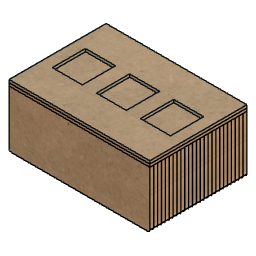
speacker-prototype1 (Autodesk Fusion 360 design; units mm, degrees)
Autodesk Fusion 360 part; units mm, degrees
(part 1 of 2)
sketch "スケッチ1" plane through (0, 0, 0) normal (0, 1, 0) x (1, 0, 0)
  line L0 (3, 0) -> (196.5, 0)
  line L1 (199.5, -3) -> (199.5, -80)
  line L2 (199.5, -80) -> (0, -80)
  line L3 (0, -80) -> (0, -3)
  arc A0 (3, 0) -> (0, -3) centre (3, -3) ccw
  arc A1 (199.5, -3) -> (196.5, 0) centre (196.5, -3) ccw
  line L4 (3, -74) -> (3, -6)
  line L5 (193.5, -77) -> (6, -77)
  line L6 (196.5, -6) -> (196.5, -74)
  line L7 (6, -3) -> (193.5, -3)
  arc A2 (3, -74) -> (6, -77) centre (6, -74) ccw
  arc A3 (6, -3) -> (3, -6) centre (6, -6) ccw
  arc A4 (193.5, -77) -> (196.5, -74) centre (193.5, -74) ccw
  arc A5 (196.5, -6) -> (193.5, -3) centre (193.5, -6) ccw
  line L8 (190.5, -74) -> (9, -74)
  line L9 (193.5, -9) -> (193.5, -71)
  line L10 (9, -6) -> (190.5, -6)
  line L11 (6, -71) -> (6, -9)
  arc A6 (6, -71) -> (9, -74) centre (9, -71) ccw
  arc A7 (9, -6) -> (6, -9) centre (9, -9) ccw
  arc A8 (193.5, -9) -> (190.5, -6) centre (190.5, -9) ccw
  arc A9 (190.5, -74) -> (193.5, -71) centre (190.5, -71) ccw
  line L12 (187.5, -71) -> (12, -71)
  line L13 (190.5, -12) -> (190.5, -68)
  line L14 (12, -9) -> (187.5, -9)
  line L15 (9, -68) -> (9, -12)
  arc A10 (9, -68) -> (12, -71) centre (12, -68) ccw
  arc A11 (12, -9) -> (9, -12) centre (12, -12) ccw
  arc A12 (187.5, -71) -> (190.5, -68) centre (187.5, -68) ccw
  arc A13 (190.5, -12) -> (187.5, -9) centre (187.5, -12) ccw
  line L16 (184.5, -68) -> (15, -68)
  line L17 (187.5, -15) -> (187.5, -65)
  line L18 (15, -12) -> (184.5, -12)
  line L19 (12, -65) -> (12, -15)
  arc A14 (12, -65) -> (15, -68) centre (15, -65) ccw
  arc A15 (15, -12) -> (12, -15) centre (15, -15) ccw
  arc A16 (184.5, -68) -> (187.5, -65) centre (184.5, -65) ccw
  arc A17 (187.5, -15) -> (184.5, -12) centre (184.5, -15) ccw
  line L20 (181.5, -65) -> (18, -65)
  line L21 (184.5, -18) -> (184.5, -62)
  line L22 (18, -15) -> (181.5, -15)
  line L23 (15, -62) -> (15, -18)
  arc A18 (15, -62) -> (18, -65) centre (18, -62) ccw
  arc A19 (18, -15) -> (15, -18) centre (18, -18) ccw
  arc A20 (181.5, -65) -> (184.5, -62) centre (181.5, -62) ccw
  arc A21 (184.5, -18) -> (181.5, -15) centre (181.5, -18) ccw
  line L24 (178.5, -62) -> (21, -62)
  line L25 (181.5, -21) -> (181.5, -59)
  line L26 (21, -18) -> (178.5, -18)
  line L27 (18, -59) -> (18, -21)
  arc A22 (18, -59) -> (21, -62) centre (21, -59) ccw
  arc A23 (21, -18) -> (18, -21) centre (21, -21) ccw
  arc A24 (178.5, -62) -> (181.5, -59) centre (178.5, -59) ccw
  arc A25 (181.5, -21) -> (178.5, -18) centre (178.5, -21) ccw
  line L28 (175.5, -59) -> (24, -59)
  line L29 (178.5, -24) -> (178.5, -56)
  line L30 (24, -21) -> (175.5, -21)
  line L31 (21, -56) -> (21, -24)
  arc A26 (21, -56) -> (24, -59) centre (24, -56) ccw
  arc A27 (24, -21) -> (21, -24) centre (24, -24) ccw
  arc A28 (175.5, -59) -> (178.5, -56) centre (175.5, -56) ccw
  arc A29 (178.5, -24) -> (175.5, -21) centre (175.5, -24) ccw
  line L32 (172.5, -56) -> (27, -56)
  line L33 (175.5, -27) -> (175.5, -53)
  line L34 (27, -24) -> (172.5, -24)
  line L35 (24, -53) -> (24, -27)
  arc A30 (24, -53) -> (27, -56) centre (27, -53) ccw
  arc A31 (27, -24) -> (24, -27) centre (27, -27) ccw
  arc A32 (172.5, -56) -> (175.5, -53) centre (172.5, -53) ccw
  arc A33 (175.5, -27) -> (172.5, -24) centre (172.5, -27) ccw
  line L36 (169.5, -53) -> (30, -53)
  line L37 (172.5, -30) -> (172.5, -50)
  line L38 (30, -27) -> (169.5, -27)
  line L39 (27, -50) -> (27, -30)
  arc A34 (27, -50) -> (30, -53) centre (30, -50) ccw
  arc A35 (30, -27) -> (27, -30) centre (30, -30) ccw
  arc A36 (169.5, -53) -> (172.5, -50) centre (169.5, -50) ccw
  arc A37 (172.5, -30) -> (169.5, -27) centre (169.5, -30) ccw
  line L40 (166.5, -50) -> (33, -50)
  line L41 (169.5, -33) -> (169.5, -47)
  line L42 (33, -30) -> (166.5, -30)
  line L43 (30, -47) -> (30, -33)
  arc A38 (30, -47) -> (33, -50) centre (33, -47) ccw
  arc A39 (33, -30) -> (30, -33) centre (33, -33) ccw
  arc A40 (166.5, -50) -> (169.5, -47) centre (166.5, -47) ccw
  arc A41 (169.5, -33) -> (166.5, -30) centre (166.5, -33) ccw
  line L44 (163.5, -47) -> (36, -47)
  line L45 (166.5, -36) -> (166.5, -44)
  line L46 (36, -33) -> (163.5, -33)
  line L47 (33, -44) -> (33, -36)
  arc A42 (33, -44) -> (36, -47) centre (36, -44) ccw
  arc A43 (36, -33) -> (33, -36) centre (36, -36) ccw
  arc A44 (163.5, -47) -> (166.5, -44) centre (163.5, -44) ccw
  arc A45 (166.5, -36) -> (163.5, -33) centre (163.5, -36) ccw
  line L48 (160.5, -44) -> (39, -44)
  line L49 (163.5, -39) -> (163.5, -41)
  line L50 (39, -36) -> (160.5, -36)
  line L51 (36, -41) -> (36, -39)
  arc A46 (36, -41) -> (39, -44) centre (39, -41) ccw
  arc A47 (39, -36) -> (36, -39) centre (39, -39) ccw
  arc A48 (160.5, -44) -> (163.5, -41) centre (160.5, -41) ccw
  arc A49 (163.5, -39) -> (160.5, -36) centre (160.5, -39) ccw
  line L52 (160.5, -41) -> (39, -41)
  line L53 (160.5, -39) -> (160.5, -41)
  line L54 (39, -39) -> (160.5, -39)
  line L55 (39, -41) -> (39, -39)
  point P0 (199.5, 0)
  dimension "d1" = 199.5
  dimension "d2" = 80
  dimension "d3" = 3
  dimension "d4" = 3
  dimension "d6" = 3
  dimension "d7" = 3
  dimension "d8" = 3
  dimension "d9" = 3
  dimension "d11" = 3
  dimension "d12" = 3
  dimension "d13" = 3
  dimension "d15" = 3
  dimension "d16" = 3
  dimension "d17" = 3
  dimension "d18" = 3
  dimension "d20" = 3
  dimension "d21" = 3
  dimension "d22" = 3
  dimension "d23" = 3
  dimension "d25" = 3
  dimension "d26" = 3
  dimension "d27" = 3
  dimension "d28" = 3
  dimension "d30" = 3
  dimension "d31" = 3
  dimension "d32" = 3
  dimension "d33" = 3
  dimension "d35" = 3
  dimension "d36" = 3
  dimension "d37" = 3
  dimension "d38" = 3
  dimension "d40" = 3
  dimension "d41" = 3
  dimension "d42" = 3
  dimension "d43" = 3
  dimension "d45" = 3
  dimension "d46" = 3
  dimension "d47" = 3
  dimension "d48" = 3
  dimension "d50" = 3
  dimension "d51" = 3
  dimension "d52" = 3
  dimension "d53" = 3
  dimension "d55" = 3
  dimension "d56" = 3
  dimension "d57" = 3
  dimension "d58" = 3
  dimension "d92" = 3
  dimension "d93" = 3
  dimension "d94" = 3
  dimension "d95" = 3
  dimension "d177" = 3
  constraint horizontal L0
  constraint vertical L1
  constraint horizontal L2
  constraint vertical L3
  constraint coincident origin L3
  constraint coincident origin L0
  constraint tangent L3 A0
  constraint tangent L0 A0
  constraint coincident P0 L1
  constraint coincident P0 L0
  constraint tangent L1 A1
  constraint tangent L0 A1
  constraint tangent L5 A2
  constraint tangent L4 A2
  constraint tangent L4 A3
  constraint tangent L7 A3
  constraint tangent L5 A4
  constraint tangent L6 A4
  constraint tangent L6 A5
  constraint tangent L7 A5
  constraint tangent L8 A6
  constraint tangent L11 A6
  constraint tangent L11 A7
  constraint tangent L10 A7
  constraint equal A6 A7
  constraint tangent L10 A8
  constraint tangent L9 A8
  constraint tangent L8 A9
  constraint tangent L9 A9
  constraint tangent L12 A10
  constraint tangent L15 A10
  constraint tangent L14 A11
  constraint tangent L15 A11
  constraint tangent L12 A12
  constraint tangent L13 A12
  constraint tangent L13 A13
  constraint tangent L14 A13
  constraint tangent L16 A14
  constraint tangent L19 A14
  constraint tangent L19 A15
  constraint tangent L18 A15
  constraint tangent L16 A16
  constraint tangent L17 A16
  constraint tangent L17 A17
  constraint tangent L18 A17
  constraint tangent L20 A18
  constraint tangent L23 A18
  constraint tangent L23 A19
  constraint tangent L22 A19
  constraint tangent L20 A20
  constraint tangent L21 A20
  constraint tangent L21 A21
  constraint tangent L22 A21
  constraint tangent L24 A22
  constraint tangent L27 A22
  constraint tangent L27 A23
  constraint tangent L26 A23
  constraint tangent L24 A24
  constraint tangent L25 A24
  constraint tangent L25 A25
  constraint tangent L26 A25
  constraint tangent L28 A26
  constraint tangent L31 A26
  constraint tangent L31 A27
  constraint tangent L30 A27
  constraint tangent L28 A28
  constraint tangent L29 A28
  constraint tangent L29 A29
  constraint tangent L30 A29
  constraint tangent L32 A30
  constraint tangent L35 A30
  constraint tangent L35 A31
  constraint tangent L34 A31
  constraint tangent L32 A32
  constraint tangent L33 A32
  constraint tangent L33 A33
  constraint tangent L34 A33
  constraint tangent L36 A34
  constraint tangent L39 A34
  constraint tangent L39 A35
  constraint tangent L38 A35
  constraint tangent L36 A36
  constraint tangent L37 A36
  constraint tangent L37 A37
  constraint tangent L38 A37
  constraint tangent L40 A38
  constraint tangent L43 A38
  constraint tangent L43 A39
  constraint tangent L42 A39
  constraint tangent L40 A40
  constraint tangent L41 A40
  constraint tangent L41 A41
  constraint tangent L42 A41
  constraint tangent L44 A42
  constraint tangent L47 A42
  constraint tangent L46 A43
  constraint tangent L47 A43
  constraint tangent L44 A44
  constraint tangent L45 A44
  constraint tangent L45 A45
  constraint tangent L46 A45
  constraint tangent L48 A46
  constraint tangent L51 A46
  constraint tangent L51 A47
  constraint tangent L50 A47
  constraint tangent L48 A48
  constraint tangent L49 A48
  constraint tangent L49 A49
  constraint tangent L50 A49
  measures "d1" distance of origin P0
  measures "d2" distance of origin L2.end
  measures "d3" radius of A0
  measures "d4" radius of A1
  measures "d6" radius of A2
  measures "d7" radius of A3
  measures "d8" radius of A4
  measures "d9" radius of A5
  measures "d11" radius of A6
  measures "d12" radius of A8
  measures "d13" radius of A9
  measures "d15" radius of A10
  measures "d16" radius of A11
  measures "d17" radius of A12
  measures "d18" radius of A13
  measures "d20" radius of A14
  measures "d21" radius of A15
  measures "d22" radius of A16
  measures "d23" radius of A17
  measures "d25" radius of A18
  measures "d26" radius of A19
  measures "d27" radius of A20
  measures "d28" radius of A21
  measures "d30" radius of A22
  measures "d31" radius of A23
  measures "d32" radius of A24
  measures "d33" radius of A25
  measures "d35" radius of A26
  measures "d36" radius of A27
  measures "d37" radius of A28
  measures "d38" radius of A29
  measures "d40" radius of A30
  measures "d41" radius of A31
  measures "d42" radius of A32
  measures "d43" radius of A33
  measures "d45" radius of A34
  measures "d46" radius of A35
  measures "d47" radius of A36
  measures "d48" radius of A37
  measures "d50" radius of A38
  measures "d51" radius of A39
  measures "d52" radius of A40
  measures "d53" radius of A41
  measures "d55" radius of A42
  measures "d56" radius of A43
  measures "d57" radius of A44
  measures "d58" radius of A45
  measures "d92" radius of A46
  measures "d93" radius of A47
  measures "d94" radius of A48
  measures "d95" radius of A49
extrude "押し出し1" add sketch "スケッチ1" against normal blind 5.5 contours L0 L1 L2 L3 A0 A1 makes body 1
extrude "押し出し2" add sketch "スケッチ1" against normal blind 5.5 from surface at -5.5 separate body contours L0 L1 L2 L3 A0 A1 | L4 L5 L6 L7 A2 A3 A4 A5 makes body 2
extrude "押し出し3" add sketch "スケッチ1" against normal blind 5.5 from surface at -11 separate body contours L0 L1 L2 L3 A0 A1 | L4 L5 L6 L7 A2 A3 A4 A5 | L8 L9 L10 L11 A6 A7 A8 A9 makes body 3
extrude "押し出し4" add sketch "スケッチ1" against normal blind 5.5 from surface at -16.5 separate body contours L0 L1 L2 L3 A0 A1 | L4 L5 L6 L7 A2 A3 A4 A5 | L8 L9 L10 L11 A6 A7 A8 A9 | L12 L13 L14 L15 A10 A11 A12 A13 makes body 4
extrude "押し出し5" add sketch "スケッチ1" against normal blind 5.5 from surface at -22 separate body contours L0 L1 L2 L3 A0 A1 | L4 L5 L6 L7 A2 A3 A4 A5 | L8 L9 L10 L11 A6 A7 A8 A9 | L12 L13 L14 L15 A10 A11 A12 A13 | L16 L17 L18 L19 A14 A15 A16 A17 makes body 5
extrude "押し出し6" add sketch "スケッチ1" against normal blind 5.5 from surface at -27.5 separate body contours L0 L1 L2 L3 A0 A1 | L4 L5 L6 L7 A2 A3 A4 A5 | L8 L9 L10 L11 A6 A7 A8 A9 | L12 L13 L14 L15 A10 A11 A12 A13 | L16 L17 L18 L19 A14 A15 A16 A17 | L20 L21 L22 L23 A18 A19 A20 A21 makes body 6
extrude "押し出し7" add sketch "スケッチ1" against normal blind 5.5 from surface at -33 separate body contours L0 L1 L2 L3 A0 A1 | L4 L5 L6 L7 A2 A3 A4 A5 | L8 L9 L10 L11 A6 A7 A8 A9 | L12 L13 L14 L15 A10 A11 A12 A13 | L16 L17 L18 L19 A14 A15 A16 A17 | L20 L21 L22 L23 A18 A19 A20 A21 | L24 L25 L26 L27 A22 A23 A24 A25 makes body 7
extrude "押し出し8" add sketch "スケッチ1" against normal blind 5.5 from surface at -38.5 separate body contours L0 L1 L2 L3 A0 A1 | L4 L5 L6 L7 A2 A3 A4 A5 | L8 L9 L10 L11 A6 A7 A8 A9 | L12 L13 L14 L15 A10 A11 A12 A13 | L16 L17 L18 L19 A14 A15 A16 A17 | L20 L21 L22 L23 A18 A19 A20 A21 | L24 L25 L26 L27 A22 A23 A24 A25 | L28 L29 L30 L31 A26 A27 A28 A29 makes body 8
extrude "押し出し9" add sketch "スケッチ1" against normal blind 5.5 from surface at -44 separate body contours L0 L1 L2 L3 A0 A1 | L4 L5 L6 L7 A2 A3 A4 A5 | L8 L9 L10 L11 A6 A7 A8 A9 | L12 L13 L14 L15 A10 A11 A12 A13 | L16 L17 L18 L19 A14 A15 A16 A17 | L20 L21 L22 L23 A18 A19 A20 A21 | L24 L25 L26 L27 A22 A23 A24 A25 | L28 L29 L30 L31 A26 A27 A28 A29 | L32 L33 L34 L35 A30 A31 A32 A33 makes body 9
extrude "押し出し10" add sketch "スケッチ1" against normal blind 5.5 from surface at -49.5 separate body contours L0 L1 L2 L3 A0 A1 | L4 L5 L6 L7 A2 A3 A4 A5 | L8 L9 L10 L11 A6 A7 A8 A9 | L12 L13 L14 L15 A10 A11 A12 A13 | L16 L17 L18 L19 A14 A15 A16 A17 | L20 L21 L22 L23 A18 A19 A20 A21 | L24 L25 L26 L27 A22 A23 A24 A25 | L28 L29 L30 L31 A26 A27 A28 A29 | L32 L33 L34 L35 A30 A31 A32 A33 | L36 L37 L38 L39 A34 A35 A36 A37 makes body 10
extrude "押し出し11" add sketch "スケッチ1" against normal blind 5.5 from surface at -55 separate body contours L0 L1 L2 L3 A0 A1 | L4 L5 L6 L7 A2 A3 A4 A5 | L8 L9 L10 L11 A6 A7 A8 A9 | L12 L13 L14 L15 A10 A11 A12 A13 | L16 L17 L18 L19 A14 A15 A16 A17 | L20 L21 L22 L23 A18 A19 A20 A21 | L24 L25 L26 L27 A22 A23 A24 A25 | L28 L29 L30 L31 A26 A27 A28 A29 | L32 L33 L34 L35 A30 A31 A32 A33 | L36 L37 L38 L39 A34 A35 A36 A37 | L40 L41 L42 L43 A38 A39 A40 A41 makes body 11
extrude "押し出し12" add sketch "スケッチ1" against normal blind 5.5 from surface at -60.5 separate body contours L0 L1 L2 L3 A0 A1 | L4 L5 L6 L7 A2 A3 A4 A5 | L8 L9 L10 L11 A6 A7 A8 A9 | L12 L13 L14 L15 A10 A11 A12 A13 | L16 L17 L18 L19 A14 A15 A16 A17 | L20 L21 L22 L23 A18 A19 A20 A21 | L24 L25 L26 L27 A22 A23 A24 A25 | L28 L29 L30 L31 A26 A27 A28 A29 | L32 L33 L34 L35 A30 A31 A32 A33 | L36 L37 L38 L39 A34 A35 A36 A37 | L40 L41 L42 L43 A38 A39 A40 A41 | L44 L45 L46 L47 A42 A43 A44 A45 makes body 12
extrude "押し出し13" add sketch "スケッチ1" against normal blind 5.5 from surface at -66 separate body contours L0 L1 L2 L3 A0 A1 | L4 L5 L6 L7 A2 A3 A4 A5 | L8 L9 L10 L11 A6 A7 A8 A9 | L12 L13 L14 L15 A10 A11 A12 A13 | L16 L17 L18 L19 A14 A15 A16 A17 | L20 L21 L22 L23 A18 A19 A20 A21 | L24 L25 L26 L27 A22 A23 A24 A25 | L28 L29 L30 L31 A26 A27 A28 A29 | L32 L33 L34 L35 A30 A31 A32 A33 | L36 L37 L38 L39 A34 A35 A36 A37 | L40 L41 L42 L43 A38 A39 A40 A41 | L44 L45 L46 L47 A42 A43 A44 A45 | L48 L49 L50 L51 A46 A47 A48 A49 | L52 L53 L54 L55 makes body 13
extrude "押し出し14" add 1 faces at (67.5, -71.5, 53.3333) along direction (0, -1, 0) blind 5.5 separate body on bodies 13 makes body 14
extrude "押し出し15" add 1 faces at (67.5, -77, 53.3333) along direction (0, -1, 0) blind 5.5 separate body on bodies 14 makes body 15
extrude "押し出し16" add 1 faces at (67.5, -82.5, 53.3333) along direction (0, -1, 0) blind 5.5 separate body on bodies 15 makes body 16
extrude "押し出し17" add 1 faces at (67.5, -88, 53.3333) along direction (0, -1, 0) blind 5.5 separate body on bodies 16 makes body 17
extrude "押し出し18" add 1 faces at (67.5, -93.5, 53.3333) along direction (0, -1, 0) blind 5.5 separate body on bodies 17 makes body 18
sketch "スケッチ2" plane through (0, -99, 0) normal (0, -1, 0) x (1, 0, 0)
  arc A0 (196.5, 0) -> (199.5, 3) centre (196.5, 3) ccw
  line L0 (199.5, 3) -> (199.5, 80)
  line L1 (199.5, 80) -> (0, 80)
  line L2 (0, 80) -> (0, 3)
  arc A1 (0, 3) -> (3, 0) centre (3, 3) ccw
  line L3 (3, 0) -> (196.5, 0)
extrude "押し出し19" add sketch "スケッチ2" along normal blind 5.5 separate body makes body 19
extrude "押し出し20" add 1 faces at (67.5, -104.5, 53.3333) along direction (0, -1, 0) blind 5.5 separate body on bodies 19 makes body 20
extrude "押し出し21" add 1 faces at (67.5, -110, 53.3333) along direction (0, -1, 0) blind 5.5 separate body on bodies 20 makes body 21
extrude "押し出し22" add 1 faces at (67.5, -115.5, 53.3333) along direction (0, -1, 0) blind 5.5 separate body on bodies 21 makes body 22
extrude "押し出し23" add 1 faces at (67.5, -121, 53.3333) along direction (0, -1, 0) blind 5.5 separate body on bodies 22 makes body 23
extrude "押し出し24" add 1 faces at (67.5, -126.5, 53.3333) along direction (0, -1, 0) blind 5.5 separate body on bodies 23 makes body 24
extrude "押し出し25" add 1 faces at (67.5, -132, 53.3333) along direction (0, -1, 0) blind 5.5 separate body on bodies 24 makes body 25
sketch "スケッチ3" plane through (0, 0, 80) normal (0, 0, 1) x (-1, 0, 0)
  line L0 (-199.5, 110) -> (0, 110)
  line L1 (0, 110) -> (0, 115.5)
  line L2 (0, 115.5) -> (-199.5, 115.5)
  line L3 (-199.5, 115.5) -> (-199.5, 110)
  line L4 (-199.5, 137.5) -> (0, 137.5)
  line L5 (-199.5, 0) -> (0, 0)
  line L6 (-199.5, 137.5) -> (0, 137.5)
  line L7 (0, 137.5) -> (0, 0)
  line L8 (0, 0) -> (-199.5, 0)
  line L9 (-199.5, 0) -> (-199.5, 137.5)
  line L10 (-194, 5.5) -> (-194, 132)
  line L11 (-194, 132) -> (-5.5, 132)
  line L12 (-5.5, 132) -> (-5.5, 5.5)
  line L13 (-5.5, 5.5) -> (-194, 5.5)
  line L14 (-11, 11) -> (-188.5, 11)
  line L15 (-188.5, 11) -> (-188.5, 126.5)
  line L16 (-188.5, 126.5) -> (-11, 126.5)
  line L17 (-11, 126.5) -> (-11, 11)
  line L18 (-183, 121) -> (-16.5, 121)
  line L19 (-16.5, 121) -> (-16.5, 16.5)
  line L20 (-16.5, 16.5) -> (-183, 16.5)
  line L21 (-183, 16.5) -> (-183, 121)
  line L22 (-177.5, 115.5) -> (-22, 115.5)
  line L23 (-22, 115.5) -> (-22, 22)
  line L24 (-22, 22) -> (-177.5, 22)
  line L25 (-177.5, 22) -> (-177.5, 115.5)
  line L26 (-172, 110) -> (-27.5, 110)
  line L27 (-27.5, 110) -> (-27.5, 27.5)
  line L28 (-27.5, 27.5) -> (-172, 27.5)
  line L29 (-172, 27.5) -> (-172, 110)
  line L30 (-166.5, 104.5) -> (-33, 104.5)
  line L31 (-33, 104.5) -> (-33, 33)
  line L32 (-33, 33) -> (-166.5, 33)
  line L33 (-166.5, 33) -> (-166.5, 104.5)
  line L34 (-161, 99) -> (-38.5, 99)
  line L35 (-38.5, 99) -> (-38.5, 38.5)
  line L36 (-38.5, 38.5) -> (-161, 38.5)
  line L37 (-161, 38.5) -> (-161, 99)
  line L38 (-44, 44) -> (-155.5, 44)
  line L39 (-155.5, 44) -> (-155.5, 93.5)
  line L40 (-155.5, 93.5) -> (-44, 93.5)
  line L41 (-44, 93.5) -> (-44, 44)
  line L42 (-150, 88) -> (-49.5, 88)
  line L43 (-49.5, 88) -> (-49.5, 49.5)
  line L44 (-49.5, 49.5) -> (-150, 49.5)
  line L45 (-150, 49.5) -> (-150, 88)
  line L46 (-55, 55) -> (-144.5, 55)
  line L47 (-144.5, 55) -> (-144.5, 82.5)
  line L48 (-144.5, 82.5) -> (-55, 82.5)
  line L49 (-55, 82.5) -> (-55, 55)
  line L50 (-139, 77) -> (-60.5, 77)
  line L51 (-60.5, 77) -> (-60.5, 60.5)
  line L52 (-60.5, 60.5) -> (-139, 60.5)
  line L53 (-139, 60.5) -> (-139, 77)
  point P0 (0, 137.5)
  dimension "d127" = 5.5
  dimension "d130" = 11
  dimension "d131" = 16.5
  dimension "d132" = 22
  dimension "d133" = 27.5
  dimension "d134" = 33
  dimension "d135" = 38.5
  dimension "d136" = 44
  dimension "d137" = 49.5
  dimension "d138" = 55
  dimension "d139" = 60.5
  constraint horizontal L6
  constraint vertical L7
  constraint horizontal L8
  constraint vertical L9
  constraint coincident L5.end L7.end
  constraint coincident L4.start L6.start
extrude "押し出し26" cut sketch "スケッチ3" against normal blind 3 contours L0 L2 L22 L23 L25 L26 | L0 L23 L24 L25 L27 L28 L29 | L0 L26 L27 L28 L29 | L0 L19 L20 L21 L23 L24 L25 | L0 L2 L21 L25 | L0 L2 L19 L23 | L0 L14 L15 L17 L19 L20 L21 | L0 L2 L15 L21 | L2 L18 L19 L21 L22 | L0 L2 L17 L19 | L0 L10 L12 L13 L14 L15 L17 | L0 L2 L10 L15 | L2 L15 L16 L17 L18 L19 L21 | L0 L2 L12 L17 | L2 L10 L11 L12 L15 L16 L17 | L30 L31 L32 L33 | L34 L35 L36 L37 | L38 L39 L40 L41 | L42 L43 L44 L45 | L46 L47 L48 L49 | L50 L51 L52 L53 bodies 2 3 4 5 6 7 8 9 10 11 12 13 14 15 16 17 18 19 20 21 22 23 24
extrude "押し出し27" cut sketch "スケッチ3" against normal blind 6 contours L0 L2 L22 L23 L25 L26 | L0 L23 L24 L25 L27 L28 L29 | L0 L26 L27 L28 L29 | L0 L19 L20 L21 L23 L24 L25 | L0 L2 L21 L25 | L0 L2 L19 L23 | L0 L14 L15 L17 L19 L20 L21 | L0 L2 L15 L21 | L2 L18 L19 L21 L22 | L0 L2 L17 L19 | L2 L15 L16 L17 L18 L19 L21 | L30 L31 L32 L33 | L34 L35 L36 L37 | L38 L39 L40 L41 | L42 L43 L44 L45 | L46 L47 L48 L49 | L50 L51 L52 L53 bodies 3 4 5 6 7 8 9 10 11 12 13 14 15 16 17 18 19 20 21 22 23
extrude "押し出し28" cut sketch "スケッチ3" against normal blind 9 contours L0 L2 L22 L23 L25 L26 | L0 L23 L24 L25 L27 L28 L29 | L0 L26 L27 L28 L29 | L0 L19 L20 L21 L23 L24 L25 | L0 L2 L21 L25 | L2 L18 L19 L21 L22 | L30 L31 L32 L33 | L34 L35 L36 L37 | L38 L39 L40 L41 | L42 L43 L44 L45 | L46 L47 L48 L49 | L50 L51 L52 L53 bodies 4 5 6 7 8 9 10 11 12 13 14 15 16 17 18 19 20 21 22
extrude "押し出し29" cut sketch "スケッチ3" against normal blind 12 contours L0 L2 L22 L23 L25 L26 | L0 L23 L24 L25 L27 L28 L29 | L0 L26 L27 L28 L29 | L30 L31 L32 L33 | L34 L35 L36 L37 | L38 L39 L40 L41 | L42 L43 L44 L45 | L46 L47 L48 L49 | L50 L51 L52 L53 bodies 5 6 7 8 9 10 11 12 13 14 15 16 17 18 19 20 21
extrude "押し出し30" cut sketch "スケッチ3" against normal blind 15 contours L0 L26 L27 L28 L29 | L30 L31 L32 L33 | L34 L35 L36 L37 | L38 L39 L40 L41 | L42 L43 L44 L45 | L46 L47 L48 L49 | L50 L51 L52 L53 bodies 6 7 8 9 10 11 12 13 14 15 16 17 18 19 20
extrude "押し出し31" cut sketch "スケッチ3" against normal blind 18 contours L30 L31 L32 L33 | L34 L35 L36 L37 | L38 L39 L40 L41 | L42 L43 L44 L45 | L46 L47 L48 L49 | L50 L51 L52 L53 bodies 7 8 9 10 11 12 13 14 15 16 17 18 19
extrude "押し出し32" cut sketch "スケッチ3" against normal blind 21 contours L34 L35 L36 L37 | L38 L39 L40 L41 | L42 L43 L44 L45 | L46 L47 L48 L49 | L50 L51 L52 L53 bodies 8 9 10 11 12 13 14 15 16 17 18
extrude "押し出し33" cut sketch "スケッチ3" against normal blind 24 contours L38 L39 L40 L41 | L42 L43 L44 L45 | L46 L47 L48 L49 | L50 L51 L52 L53 bodies 9 10 11 12 13 14 15 16 17
sketch "スケッチ4" plane through (22, 0, 0) normal (1, 0, 0) x (0, 1, 0)
  line L0 (-110, 74) -> (-115.5, 74)
  line L1 (-115.5, 74) -> (-115.5, 68)
  line L2 (-115.5, 68) -> (-110, 68)
  line L3 (-110, 68) -> (-110, 74)
  line L4 (-115.5, 71) -> (-110, 71)
  constraint midpoint L1 L4.start
  constraint midpoint L3 L4.end
extrude "押し出し34" cut sketch "スケッチ4" against normal blind 5.5 contours L0 L1 L3 L4 bodies 21
extrude "押し出し35" cut sketch "スケッチ3" against normal blind 27 contours L42 L43 L44 L45 | L46 L47 L48 L49 | L50 L51 L52 L53 bodies 10 11 12 13 14 15 16
extrude "押し出し36" cut sketch "スケッチ3" against normal blind 30 contours L46 L47 L48 L49 | L50 L51 L52 L53 bodies 11 12 13 14 15
extrude "押し出し37" cut sketch "スケッチ3" against normal blind 33 contours L50 L51 L52 L53 bodies 12 13 14
extrude "押し出し38" cut 1 faces at (86.6667, -67.8333, 47) along direction (0, 0, -1) blind 3 on bodies 13 bodies 13
extrude "押し出し39" add sketch "スケッチ3" along normal blind 4 separate body contours L0 L2 L22 L23 L25 L26 | L0 L23 L24 L25 L27 L28 L29 | L0 L26 L27 L28 L29 | L0 L19 L20 L21 L23 L24 L25 | L0 L2 L21 L25 | L0 L2 L19 L23 | L0 L14 L15 L17 L19 L20 L21 | L0 L2 L15 L21 | L2 L18 L19 L21 L22 | L0 L2 L17 L19 | L0 L10 L12 L13 L14 L15 L17 | L0 L2 L10 L15 | L2 L15 L16 L17 L18 L19 L21 | L0 L2 L12 L17 | L0 L5 L7 L8 L9 L10 L12 L13 | L0 L2 L3 L9 L10 | L2 L10 L11 L12 L15 L16 L17 | L0 L1 L2 L7 L12 | L2 L4 L6 L7 L9 L10 L11 L12 | L30 L31 L32 L33 | L34 L35 L36 L37 | L38 L39 L40 L41 | L42 L43 L44 L45 | L46 L47 L48 L49 | L50 L51 L52 L53 makes body 26
extrude "押し出し40" add 1 faces at (133, -73.3333, 84) along direction (0, 0, 1) blind 4 separate body on bodies 26 makes body 27
ref_plane "作業平面1" through (99.75, -68.75, 88) normal (0, 0, 1) x (1, 0, 0)
sketch "スケッチ5" plane through (0, 0, 80) normal (0, 0, 1) x (-1, 0, 0)
  line L0 (-199.5, 137.5) -> (0, 0) construction
  line L1 (0, 137.5) -> (-199.5, 0) construction
  line L2 (-78.5, 45.25) -> (-121, 45.25)
  line L3 (-121, 45.25) -> (-121, 92.25)
  line L4 (-121, 92.25) -> (-78.5, 92.25)
  line L5 (-78.5, 92.25) -> (-78.5, 45.25)
  line L6 (-78.5, 45.25) -> (-121, 92.25) construction
  line L7 (-121, 45.25) -> (-78.5, 92.25) construction
  line L8 (-58.5, 92.25) -> (-16, 92.25)
  line L9 (-16, 92.25) -> (-16, 45.25)
  line L10 (-16, 45.25) -> (-58.5, 45.25)
  line L11 (-58.5, 45.25) -> (-58.5, 92.25)
  line L12 (-99.75, 92.25) -> (-99.75, 45.25) construction
  line L13 (-183.5, 92.25) -> (-183.5, 45.25)
  line L14 (-183.5, 45.25) -> (-141, 45.25)
  line L15 (-141, 92.25) -> (-183.5, 92.25)
  line L16 (-141, 45.25) -> (-141, 92.25)
  point P0 (-199.5, 137.5)
  point P1 (0, 137.5)
  point P2 (-199.5, 0)
  point P3 (-99.75, 68.75)
  point P4 (-99.75, 68.75)
  dimension "d169" = 42.5
  dimension "d170" = 47
  dimension "d171" = 42.5
  dimension "d172" = 47
  dimension "d173" = 20
  constraint coincident P0 L0.start
  constraint coincident L0.end origin
  constraint coincident P1 L1.start
  constraint coincident P2 L1.end
  constraint midpoint L0 P4
  constraint horizontal L2
  constraint perpendicular L2 L3
  constraint parallel L2 L4
  constraint parallel L3 L5
  constraint coincident L6 P4
  constraint coincident L7 P4
  constraint coincident P4 P3
  constraint horizontal L8
  constraint vertical L9
  constraint horizontal L10
  constraint vertical L11
  constraint midpoint L4 L12.start
  constraint midpoint L2 L12.end
  constraint symmetric L8.start L12 L15.start
  constraint symmetric L8.end L12 L13.start
  constraint symmetric L9.end L12 L13.end
  constraint symmetric L10.end L12 L14.end
  measures "d169" distance of L3.end L4.end
  measures "d170" distance of L2.end L3.end
  measures "d171" distance of L8.start L8.end
  measures "d172" distance of L8.start L10.end
  measures "d173" distance of L5 L11
extrude "押し出し41" cut sketch "スケッチ5" along normal blind 4 from surface at 4 bodies 27
extrude "押し出し42" cut sketch "スケッチ1" against normal blind 71.5 contours L52 L53 L54 L55 bodies 13
extrude "押し出し43" cut 1 faces at (86.6667, -67.8333, 44) along direction (0, 0, -1) blind 3 on bodies 13 bodies 13
sketch "スケッチ6" plane through (0, 0, 88) normal (0, 0, 1) x (-1, 0, 0)
  line L0 (-183.5, 45.25) -> (-183.5, 92.25)
  line L1 (-183.5, 92.25) -> (-141, 92.25)
  line L2 (-141, 92.25) -> (-141, 45.25)
  line L3 (-141, 45.25) -> (-183.5, 45.25)
  line L4 (-78.5, 45.25) -> (-121, 45.25)
  line L5 (-121, 45.25) -> (-121, 92.25)
  line L6 (-121, 92.25) -> (-78.5, 92.25)
  line L7 (-78.5, 92.25) -> (-78.5, 45.25)
  line L8 (-58.5, 92.25) -> (-16, 92.25)
  line L9 (-16, 92.25) -> (-16, 45.25)
  line L10 (-16, 45.25) -> (-58.5, 45.25)
  line L11 (-58.5, 45.25) -> (-58.5, 92.25)
  line L12 (-199.5, 0) -> (0, 0)
  line L13 (0, 0) -> (0, 137.5)
  line L14 (0, 137.5) -> (-199.5, 137.5)
  line L15 (-199.5, 137.5) -> (-199.5, 0)
sketch "スケッチ7" plane through (0, 0, 0) normal (0, 1, 0) x (-1, 0, 0)
  arc A0 (-193.5, 77) -> (-196.5, 74) centre (-193.5, 74) ccw
  line L0 (-193.5, 77) -> (-6, 77)
  arc A1 (-3, 74) -> (-6, 77) centre (-6, 74) ccw
  line L1 (-3, 74) -> (-3, 6)
  arc A2 (-6, 3) -> (-3, 6) centre (-6, 6) ccw
  line L2 (-6, 3) -> (-193.5, 3)
  arc A3 (-196.5, 6) -> (-193.5, 3) centre (-193.5, 6) ccw
  line L3 (-196.5, 6) -> (-196.5, 74)
  line L4 (-199.5, 80) -> (-199.5, 3)
  arc A4 (-199.5, 3) -> (-196.5, 0) centre (-196.5, 3) ccw
  line L5 (-196.5, 0) -> (-3, 0)
  arc A5 (-3, 0) -> (0, 3) centre (-3, 3) ccw
  line L6 (0, 3) -> (0, 80)
  line L7 (0, 80) -> (-199.5, 80)
sketch "スケッチ8" plane through (0, -5.5, 0) normal (0, 1, 0) x (-1, 0, 0)
  line L0 (-5.5, 80) -> (-5.5, 77)
  line L1 (-5.5, 77) -> (-194, 77)
  line L2 (-194, 77) -> (-194, 80)
  line L3 (-194, 80) -> (-199.5, 80)
  line L4 (-199.5, 80) -> (-199.5, 3)
  arc A0 (-199.5, 3) -> (-196.5, 0) centre (-196.5, 3) ccw
  line L5 (-196.5, 0) -> (-3, 0)
  arc A1 (-3, 0) -> (0, 3) centre (-3, 3) ccw
  line L6 (0, 3) -> (0, 80)
  line L7 (0, 80) -> (-5.5, 80)
  line L8 (-6, 71) -> (-6, 9)
  arc A2 (-9, 6) -> (-6, 9) centre (-9, 9) ccw
  line L9 (-9, 6) -> (-190.5, 6)
  arc A3 (-193.5, 9) -> (-190.5, 6) centre (-190.5, 9) ccw
  line L10 (-193.5, 9) -> (-193.5, 71)
  arc A4 (-190.5, 74) -> (-193.5, 71) centre (-190.5, 71) ccw
  line L11 (-190.5, 74) -> (-9, 74)
  arc A5 (-6, 71) -> (-9, 74) centre (-9, 71) ccw
sketch "スケッチ9" plane through (0, -11, 0) normal (0, 1, 0) x (-1, 0, 0)
  line L0 (-187.5, 71) -> (-12, 71)
  arc A0 (-9, 68) -> (-12, 71) centre (-12, 68) ccw
  line L1 (-9, 68) -> (-9, 12)
  arc A1 (-12, 9) -> (-9, 12) centre (-12, 12) ccw
  line L2 (-12, 9) -> (-187.5, 9)
  arc A2 (-190.5, 12) -> (-187.5, 9) centre (-187.5, 12) ccw
  line L3 (-190.5, 12) -> (-190.5, 68)
  arc A3 (-187.5, 71) -> (-190.5, 68) centre (-187.5, 68) ccw
  line L4 (-11, 77) -> (-11, 74)
  line L5 (-11, 74) -> (-188.5, 74)
  line L6 (-188.5, 74) -> (-188.5, 77)
  line L7 (-188.5, 77) -> (-194, 77)
  line L8 (-194, 77) -> (-194, 80)
  line L9 (-194, 80) -> (-199.5, 80)
  line L10 (-199.5, 80) -> (-199.5, 3)
  arc A4 (-199.5, 3) -> (-196.5, 0) centre (-196.5, 3) ccw
  line L11 (-196.5, 0) -> (-3, 0)
  arc A5 (-3, 0) -> (0, 3) centre (-3, 3) ccw
  line L12 (0, 3) -> (0, 80)
  line L13 (0, 80) -> (-5.5, 80)
  line L14 (-5.5, 80) -> (-5.5, 77)
  line L15 (-5.5, 77) -> (-11, 77)
sketch "スケッチ10" plane through (0, -16.5, 0) normal (0, 1, 0) x (-1, 0, 0)
  line L0 (-184.5, 68) -> (-15, 68)
  arc A0 (-12, 65) -> (-15, 68) centre (-15, 65) ccw
  line L1 (-12, 65) -> (-12, 15)
  arc A1 (-15, 12) -> (-12, 15) centre (-15, 15) ccw
  line L2 (-15, 12) -> (-184.5, 12)
  arc A2 (-187.5, 15) -> (-184.5, 12) centre (-184.5, 15) ccw
  line L3 (-187.5, 15) -> (-187.5, 65)
  arc A3 (-184.5, 68) -> (-187.5, 65) centre (-184.5, 65) ccw
  line L4 (-16.5, 74) -> (-16.5, 71)
  line L5 (-16.5, 71) -> (-183, 71)
  line L6 (-183, 71) -> (-183, 74)
  line L7 (-183, 74) -> (-188.5, 74)
  line L8 (-188.5, 74) -> (-188.5, 77)
  line L9 (-188.5, 77) -> (-194, 77)
  line L10 (-194, 77) -> (-194, 80)
  line L11 (-194, 80) -> (-199.5, 80)
  line L12 (-199.5, 80) -> (-199.5, 3)
  arc A4 (-199.5, 3) -> (-196.5, 0) centre (-196.5, 3) ccw
  line L13 (-196.5, 0) -> (-3, 0)
  arc A5 (-3, 0) -> (0, 3) centre (-3, 3) ccw
  line L14 (0, 3) -> (0, 80)
  line L15 (0, 80) -> (-5.5, 80)
  line L16 (-5.5, 80) -> (-5.5, 77)
  line L17 (-5.5, 77) -> (-11, 77)
  line L18 (-11, 77) -> (-11, 74)
  line L19 (-11, 74) -> (-16.5, 74)
sketch "スケッチ11" plane through (0, -22, 0) normal (0, 1, 0) x (-1, 0, 0)
  line L0 (-181.5, 65) -> (-18, 65)
  arc A0 (-15, 62) -> (-18, 65) centre (-18, 62) ccw
  line L1 (-15, 62) -> (-15, 18)
  arc A1 (-18, 15) -> (-15, 18) centre (-18, 18) ccw
  line L2 (-18, 15) -> (-181.5, 15)
  arc A2 (-184.5, 18) -> (-181.5, 15) centre (-181.5, 18) ccw
  line L3 (-184.5, 18) -> (-184.5, 62)
  arc A3 (-181.5, 65) -> (-184.5, 62) centre (-181.5, 62) ccw
  line L4 (-22, 71) -> (-22, 68)
  line L5 (-22, 68) -> (-177.5, 68)
  line L6 (-177.5, 68) -> (-177.5, 71)
  line L7 (-177.5, 71) -> (-183, 71)
  line L8 (-183, 71) -> (-183, 74)
  line L9 (-183, 74) -> (-188.5, 74)
  line L10 (-188.5, 74) -> (-188.5, 77)
  line L11 (-188.5, 77) -> (-194, 77)
  line L12 (-194, 77) -> (-194, 80)
  line L13 (-194, 80) -> (-199.5, 80)
  line L14 (-199.5, 80) -> (-199.5, 3)
  arc A4 (-199.5, 3) -> (-196.5, 0) centre (-196.5, 3) ccw
  line L15 (-196.5, 0) -> (-3, 0)
  arc A5 (-3, 0) -> (0, 3) centre (-3, 3) ccw
  line L16 (0, 3) -> (0, 80)
  line L17 (0, 80) -> (-5.5, 80)
  line L18 (-5.5, 80) -> (-5.5, 77)
  line L19 (-5.5, 77) -> (-11, 77)
  line L20 (-11, 77) -> (-11, 74)
  line L21 (-11, 74) -> (-16.5, 74)
  line L22 (-16.5, 74) -> (-16.5, 71)
  line L23 (-16.5, 71) -> (-22, 71)
sketch "スケッチ12" plane through (0, -27.5, 0) normal (0, 1, 0) x (-1, 0, 0)
  line L0 (-27.5, 68) -> (-27.5, 65)
  line L1 (-27.5, 65) -> (-172, 65)
  line L2 (-172, 65) -> (-172, 68)
  line L3 (-172, 68) -> (-177.5, 68)
  line L4 (-177.5, 68) -> (-177.5, 71)
  line L5 (-177.5, 71) -> (-183, 71)
  line L6 (-183, 71) -> (-183, 74)
  line L7 (-183, 74) -> (-188.5, 74)
  line L8 (-188.5, 74) -> (-188.5, 77)
  line L9 (-188.5, 77) -> (-194, 77)
  line L10 (-194, 77) -> (-194, 80)
  line L11 (-194, 80) -> (-199.5, 80)
  line L12 (-199.5, 80) -> (-199.5, 3)
  arc A0 (-199.5, 3) -> (-196.5, 0) centre (-196.5, 3) ccw
  line L13 (-196.5, 0) -> (-3, 0)
  arc A1 (-3, 0) -> (0, 3) centre (-3, 3) ccw
  line L14 (0, 3) -> (0, 80)
  line L15 (0, 80) -> (-5.5, 80)
  line L16 (-5.5, 80) -> (-5.5, 77)
  line L17 (-5.5, 77) -> (-11, 77)
  line L18 (-11, 77) -> (-11, 74)
  line L19 (-11, 74) -> (-16.5, 74)
  line L20 (-16.5, 74) -> (-16.5, 71)
  line L21 (-16.5, 71) -> (-22, 71)
  line L22 (-22, 71) -> (-22, 68)
  line L23 (-22, 68) -> (-27.5, 68)
  line L24 (-178.5, 62) -> (-21, 62)
  arc A2 (-18, 59) -> (-21, 62) centre (-21, 59) ccw
  line L25 (-18, 59) -> (-18, 21)
  arc A3 (-21, 18) -> (-18, 21) centre (-21, 21) ccw
  line L26 (-21, 18) -> (-178.5, 18)
  arc A4 (-181.5, 21) -> (-178.5, 18) centre (-178.5, 21) ccw
  line L27 (-181.5, 21) -> (-181.5, 59)
  arc A5 (-178.5, 62) -> (-181.5, 59) centre (-178.5, 59) ccw
sketch "スケッチ13" plane through (0, -33, 0) normal (0, 1, 0) x (-1, 0, 0)
  line L0 (-175.5, 59) -> (-24, 59)
  arc A0 (-21, 56) -> (-24, 59) centre (-24, 56) ccw
  line L1 (-21, 56) -> (-21, 24)
  arc A1 (-24, 21) -> (-21, 24) centre (-24, 24) ccw
  line L2 (-24, 21) -> (-175.5, 21)
  arc A2 (-178.5, 24) -> (-175.5, 21) centre (-175.5, 24) ccw
  line L3 (-178.5, 24) -> (-178.5, 56)
  arc A3 (-175.5, 59) -> (-178.5, 56) centre (-175.5, 56) ccw
  line L4 (-33, 65) -> (-33, 62)
  line L5 (-33, 62) -> (-166.5, 62)
  line L6 (-166.5, 62) -> (-166.5, 65)
  line L7 (-166.5, 65) -> (-172, 65)
  line L8 (-172, 65) -> (-172, 68)
  line L9 (-172, 68) -> (-177.5, 68)
  line L10 (-177.5, 68) -> (-177.5, 71)
  line L11 (-177.5, 71) -> (-183, 71)
  line L12 (-183, 71) -> (-183, 74)
  line L13 (-183, 74) -> (-188.5, 74)
  line L14 (-188.5, 74) -> (-188.5, 77)
  line L15 (-188.5, 77) -> (-194, 77)
  line L16 (-194, 77) -> (-194, 80)
  line L17 (-194, 80) -> (-199.5, 80)
  line L18 (-199.5, 80) -> (-199.5, 3)
  arc A4 (-199.5, 3) -> (-196.5, 0) centre (-196.5, 3) ccw
  line L19 (-196.5, 0) -> (-3, 0)
  arc A5 (-3, 0) -> (0, 3) centre (-3, 3) ccw
  line L20 (0, 3) -> (0, 80)
  line L21 (0, 80) -> (-5.5, 80)
  line L22 (-5.5, 80) -> (-5.5, 77)
  line L23 (-5.5, 77) -> (-11, 77)
  line L24 (-11, 77) -> (-11, 74)
  line L25 (-11, 74) -> (-16.5, 74)
  line L26 (-16.5, 74) -> (-16.5, 71)
  line L27 (-16.5, 71) -> (-22, 71)
  line L28 (-22, 71) -> (-22, 68)
  line L29 (-22, 68) -> (-27.5, 68)
  line L30 (-27.5, 68) -> (-27.5, 65)
  line L31 (-27.5, 65) -> (-33, 65)
sketch "スケッチ14" plane through (0, -38.5, 0) normal (0, 1, 0) x (-1, 0, 0)
  line L0 (-38.5, 62) -> (-38.5, 59)
  line L1 (-38.5, 59) -> (-161, 59)
  line L2 (-161, 59) -> (-161, 62)
  line L3 (-161, 62) -> (-166.5, 62)
  line L4 (-166.5, 62) -> (-166.5, 65)
  line L5 (-166.5, 65) -> (-172, 65)
  line L6 (-172, 65) -> (-172, 68)
  line L7 (-172, 68) -> (-177.5, 68)
  line L8 (-177.5, 68) -> (-177.5, 71)
  line L9 (-177.5, 71) -> (-183, 71)
  line L10 (-183, 71) -> (-183, 74)
  line L11 (-183, 74) -> (-188.5, 74)
  line L12 (-188.5, 74) -> (-188.5, 77)
  line L13 (-188.5, 77) -> (-194, 77)
  line L14 (-194, 77) -> (-194, 80)
  line L15 (-194, 80) -> (-199.5, 80)
  line L16 (-199.5, 80) -> (-199.5, 3)
  arc A0 (-199.5, 3) -> (-196.5, 0) centre (-196.5, 3) ccw
  line L17 (-196.5, 0) -> (-3, 0)
  arc A1 (-3, 0) -> (0, 3) centre (-3, 3) ccw
  line L18 (0, 3) -> (0, 80)
  line L19 (0, 80) -> (-5.5, 80)
  line L20 (-5.5, 80) -> (-5.5, 77)
  line L21 (-5.5, 77) -> (-11, 77)
  line L22 (-11, 77) -> (-11, 74)
  line L23 (-11, 74) -> (-16.5, 74)
  line L24 (-16.5, 74) -> (-16.5, 71)
  line L25 (-16.5, 71) -> (-22, 71)
  line L26 (-22, 71) -> (-22, 68)
  line L27 (-22, 68) -> (-27.5, 68)
  line L28 (-27.5, 68) -> (-27.5, 65)
  line L29 (-27.5, 65) -> (-33, 65)
  line L30 (-33, 65) -> (-33, 62)
  line L31 (-33, 62) -> (-38.5, 62)
  line L32 (-172.5, 56) -> (-27, 56)
  arc A2 (-24, 53) -> (-27, 56) centre (-27, 53) ccw
  line L33 (-24, 53) -> (-24, 27)
  arc A3 (-27, 24) -> (-24, 27) centre (-27, 27) ccw
  line L34 (-27, 24) -> (-172.5, 24)
  arc A4 (-175.5, 27) -> (-172.5, 24) centre (-172.5, 27) ccw
  line L35 (-175.5, 27) -> (-175.5, 53)
  arc A5 (-172.5, 56) -> (-175.5, 53) centre (-172.5, 53) ccw
sketch "スケッチ15" plane through (0, -44, 0) normal (0, 1, 0) x (-1, 0, 0)
  line L0 (-169.5, 53) -> (-30, 53)
  arc A0 (-27, 50) -> (-30, 53) centre (-30, 50) ccw
  line L1 (-27, 50) -> (-27, 30)
  arc A1 (-30, 27) -> (-27, 30) centre (-30, 30) ccw
  line L2 (-30, 27) -> (-169.5, 27)
  arc A2 (-172.5, 30) -> (-169.5, 27) centre (-169.5, 30) ccw
  line L3 (-172.5, 30) -> (-172.5, 50)
  arc A3 (-169.5, 53) -> (-172.5, 50) centre (-169.5, 50) ccw
  line L4 (-44, 59) -> (-44, 56)
  line L5 (-44, 56) -> (-155.5, 56)
  line L6 (-155.5, 56) -> (-155.5, 59)
  line L7 (-155.5, 59) -> (-161, 59)
  line L8 (-161, 59) -> (-161, 62)
  line L9 (-161, 62) -> (-166.5, 62)
  line L10 (-166.5, 62) -> (-166.5, 65)
  line L11 (-166.5, 65) -> (-172, 65)
  line L12 (-172, 65) -> (-172, 68)
  line L13 (-172, 68) -> (-177.5, 68)
  line L14 (-177.5, 68) -> (-177.5, 71)
  line L15 (-177.5, 71) -> (-183, 71)
  line L16 (-183, 71) -> (-183, 74)
  line L17 (-183, 74) -> (-188.5, 74)
  line L18 (-188.5, 74) -> (-188.5, 77)
  line L19 (-188.5, 77) -> (-194, 77)
  line L20 (-194, 77) -> (-194, 80)
  line L21 (-194, 80) -> (-199.5, 80)
  line L22 (-199.5, 80) -> (-199.5, 3)
  arc A4 (-199.5, 3) -> (-196.5, 0) centre (-196.5, 3) ccw
  line L23 (-196.5, 0) -> (-3, 0)
  arc A5 (-3, 0) -> (0, 3) centre (-3, 3) ccw
  line L24 (0, 3) -> (0, 80)
  line L25 (0, 80) -> (-5.5, 80)
  line L26 (-5.5, 80) -> (-5.5, 77)
  line L27 (-5.5, 77) -> (-11, 77)
  line L28 (-11, 77) -> (-11, 74)
  line L29 (-11, 74) -> (-16.5, 74)
  line L30 (-16.5, 74) -> (-16.5, 71)
  line L31 (-16.5, 71) -> (-22, 71)
  line L32 (-22, 71) -> (-22, 68)
  line L33 (-22, 68) -> (-27.5, 68)
  line L34 (-27.5, 68) -> (-27.5, 65)
  line L35 (-27.5, 65) -> (-33, 65)
  line L36 (-33, 65) -> (-33, 62)
  line L37 (-33, 62) -> (-38.5, 62)
  line L38 (-38.5, 62) -> (-38.5, 59)
  line L39 (-38.5, 59) -> (-44, 59)
sketch "スケッチ16" plane through (0, -49.5, 0) normal (0, 1, 0) x (-1, 0, 0)
  line L0 (-166.5, 50) -> (-33, 50)
  arc A0 (-30, 47) -> (-33, 50) centre (-33, 47) ccw
  line L1 (-30, 47) -> (-30, 33)
  arc A1 (-33, 30) -> (-30, 33) centre (-33, 33) ccw
  line L2 (-33, 30) -> (-166.5, 30)
  arc A2 (-169.5, 33) -> (-166.5, 30) centre (-166.5, 33) ccw
  line L3 (-169.5, 33) -> (-169.5, 47)
  arc A3 (-166.5, 50) -> (-169.5, 47) centre (-166.5, 47) ccw
  line L4 (-49.5, 56) -> (-49.5, 53)
  line L5 (-49.5, 53) -> (-150, 53)
  line L6 (-150, 53) -> (-150, 56)
  line L7 (-150, 56) -> (-155.5, 56)
  line L8 (-155.5, 56) -> (-155.5, 59)
  line L9 (-155.5, 59) -> (-161, 59)
  line L10 (-161, 59) -> (-161, 62)
  line L11 (-161, 62) -> (-166.5, 62)
  line L12 (-166.5, 62) -> (-166.5, 65)
  line L13 (-166.5, 65) -> (-172, 65)
  line L14 (-172, 65) -> (-172, 68)
  line L15 (-172, 68) -> (-177.5, 68)
  line L16 (-177.5, 68) -> (-177.5, 71)
  line L17 (-177.5, 71) -> (-183, 71)
  line L18 (-183, 71) -> (-183, 74)
  line L19 (-183, 74) -> (-188.5, 74)
  line L20 (-188.5, 74) -> (-188.5, 77)
  line L21 (-188.5, 77) -> (-194, 77)
  line L22 (-194, 77) -> (-194, 80)
  line L23 (-194, 80) -> (-199.5, 80)
  line L24 (-199.5, 80) -> (-199.5, 3)
  arc A4 (-199.5, 3) -> (-196.5, 0) centre (-196.5, 3) ccw
  line L25 (-196.5, 0) -> (-3, 0)
  arc A5 (-3, 0) -> (0, 3) centre (-3, 3) ccw
  line L26 (0, 3) -> (0, 80)
  line L27 (0, 80) -> (-5.5, 80)
  line L28 (-5.5, 80) -> (-5.5, 77)
  line L29 (-5.5, 77) -> (-11, 77)
  line L30 (-11, 77) -> (-11, 74)
  line L31 (-11, 74) -> (-16.5, 74)
  line L32 (-16.5, 74) -> (-16.5, 71)
  line L33 (-16.5, 71) -> (-22, 71)
  line L34 (-22, 71) -> (-22, 68)
  line L35 (-22, 68) -> (-27.5, 68)
  line L36 (-27.5, 68) -> (-27.5, 65)
  line L37 (-27.5, 65) -> (-33, 65)
  line L38 (-33, 65) -> (-33, 62)
  line L39 (-33, 62) -> (-38.5, 62)
  line L40 (-38.5, 62) -> (-38.5, 59)
  line L41 (-38.5, 59) -> (-44, 59)
  line L42 (-44, 59) -> (-44, 56)
  line L43 (-44, 56) -> (-49.5, 56)
sketch "スケッチ17" plane through (0, -55, 0) normal (0, 1, 0) x (-1, 0, 0)
  line L0 (-55, 53) -> (-55, 50)
  line L1 (-55, 50) -> (-144.5, 50)
  line L2 (-144.5, 50) -> (-144.5, 53)
  line L3 (-144.5, 53) -> (-150, 53)
  line L4 (-150, 53) -> (-150, 56)
  line L5 (-150, 56) -> (-155.5, 56)
  line L6 (-155.5, 56) -> (-155.5, 59)
  line L7 (-155.5, 59) -> (-161, 59)
  line L8 (-161, 59) -> (-161, 62)
  line L9 (-161, 62) -> (-166.5, 62)
  line L10 (-166.5, 62) -> (-166.5, 65)
  line L11 (-166.5, 65) -> (-172, 65)
  line L12 (-172, 65) -> (-172, 68)
  line L13 (-172, 68) -> (-177.5, 68)
  line L14 (-177.5, 68) -> (-177.5, 71)
  line L15 (-177.5, 71) -> (-183, 71)
  line L16 (-183, 71) -> (-183, 74)
  line L17 (-183, 74) -> (-188.5, 74)
  line L18 (-188.5, 74) -> (-188.5, 77)
  line L19 (-188.5, 77) -> (-194, 77)
  line L20 (-194, 77) -> (-194, 80)
  line L21 (-194, 80) -> (-199.5, 80)
  line L22 (-199.5, 80) -> (-199.5, 3)
  arc A0 (-199.5, 3) -> (-196.5, 0) centre (-196.5, 3) ccw
  line L23 (-196.5, 0) -> (-3, 0)
  arc A1 (-3, 0) -> (0, 3) centre (-3, 3) ccw
  line L24 (0, 3) -> (0, 80)
  line L25 (0, 80) -> (-5.5, 80)
  line L26 (-5.5, 80) -> (-5.5, 77)
  line L27 (-5.5, 77) -> (-11, 77)
  line L28 (-11, 77) -> (-11, 74)
  line L29 (-11, 74) -> (-16.5, 74)
  line L30 (-16.5, 74) -> (-16.5, 71)
  line L31 (-16.5, 71) -> (-22, 71)
  line L32 (-22, 71) -> (-22, 68)
  line L33 (-22, 68) -> (-27.5, 68)
  line L34 (-27.5, 68) -> (-27.5, 65)
  line L35 (-27.5, 65) -> (-33, 65)
  line L36 (-33, 65) -> (-33, 62)
  line L37 (-33, 62) -> (-38.5, 62)
  line L38 (-38.5, 62) -> (-38.5, 59)
  line L39 (-38.5, 59) -> (-44, 59)
  line L40 (-44, 59) -> (-44, 56)
  line L41 (-44, 56) -> (-49.5, 56)
  line L42 (-49.5, 56) -> (-49.5, 53)
  line L43 (-49.5, 53) -> (-55, 53)
  line L44 (-163.5, 47) -> (-36, 47)
  arc A2 (-33, 44) -> (-36, 47) centre (-36, 44) ccw
  line L45 (-33, 44) -> (-33, 36)
  arc A3 (-36, 33) -> (-33, 36) centre (-36, 36) ccw
  line L46 (-36, 33) -> (-163.5, 33)
  arc A4 (-166.5, 36) -> (-163.5, 33) centre (-163.5, 36) ccw
  line L47 (-166.5, 36) -> (-166.5, 44)
  arc A5 (-163.5, 47) -> (-166.5, 44) centre (-163.5, 44) ccw
sketch "スケッチ18" plane through (0, -60.5, 0) normal (0, 1, 0) x (-1, 0, 0)
  line L0 (-160.5, 44) -> (-39, 44)
  arc A0 (-36, 41) -> (-39, 44) centre (-39, 41) ccw
  line L1 (-36, 41) -> (-36, 39)
  arc A1 (-39, 36) -> (-36, 39) centre (-39, 39) ccw
  line L2 (-39, 36) -> (-160.5, 36)
  arc A2 (-163.5, 39) -> (-160.5, 36) centre (-160.5, 39) ccw
  line L3 (-163.5, 39) -> (-163.5, 41)
  arc A3 (-160.5, 44) -> (-163.5, 41) centre (-160.5, 41) ccw
  line L4 (-60.5, 50) -> (-60.5, 47)
  line L5 (-60.5, 47) -> (-139, 47)
  line L6 (-139, 47) -> (-139, 50)
  line L7 (-139, 50) -> (-144.5, 50)
  line L8 (-144.5, 50) -> (-144.5, 53)
  line L9 (-144.5, 53) -> (-150, 53)
  line L10 (-150, 53) -> (-150, 56)
  line L11 (-150, 56) -> (-155.5, 56)
  line L12 (-155.5, 56) -> (-155.5, 59)
  line L13 (-155.5, 59) -> (-161, 59)
  line L14 (-161, 59) -> (-161, 62)
  line L15 (-161, 62) -> (-166.5, 62)
  line L16 (-166.5, 62) -> (-166.5, 65)
  line L17 (-166.5, 65) -> (-172, 65)
  line L18 (-172, 65) -> (-172, 68)
  line L19 (-172, 68) -> (-177.5, 68)
  line L20 (-177.5, 68) -> (-177.5, 71)
  line L21 (-177.5, 71) -> (-183, 71)
  line L22 (-183, 71) -> (-183, 74)
  line L23 (-183, 74) -> (-188.5, 74)
  line L24 (-188.5, 74) -> (-188.5, 77)
  line L25 (-188.5, 77) -> (-194, 77)
  line L26 (-194, 77) -> (-194, 80)
  line L27 (-194, 80) -> (-199.5, 80)
  line L28 (-199.5, 80) -> (-199.5, 3)
  arc A4 (-199.5, 3) -> (-196.5, 0) centre (-196.5, 3) ccw
  line L29 (-196.5, 0) -> (-3, 0)
  arc A5 (-3, 0) -> (0, 3) centre (-3, 3) ccw
  line L30 (0, 3) -> (0, 80)
  line L31 (0, 80) -> (-5.5, 80)
  line L32 (-5.5, 80) -> (-5.5, 77)
  line L33 (-5.5, 77) -> (-11, 77)
  line L34 (-11, 77) -> (-11, 74)
  line L35 (-11, 74) -> (-16.5, 74)
  line L36 (-16.5, 74) -> (-16.5, 71)
  line L37 (-16.5, 71) -> (-22, 71)
  line L38 (-22, 71) -> (-22, 68)
  line L39 (-22, 68) -> (-27.5, 68)
  line L40 (-27.5, 68) -> (-27.5, 65)
  line L41 (-27.5, 65) -> (-33, 65)
  line L42 (-33, 65) -> (-33, 62)
  line L43 (-33, 62) -> (-38.5, 62)
  line L44 (-38.5, 62) -> (-38.5, 59)
  line L45 (-38.5, 59) -> (-44, 59)
  line L46 (-44, 59) -> (-44, 56)
  line L47 (-44, 56) -> (-49.5, 56)
  line L48 (-49.5, 56) -> (-49.5, 53)
  line L49 (-49.5, 53) -> (-55, 53)
  line L50 (-55, 53) -> (-55, 50)
  line L51 (-55, 50) -> (-60.5, 50)
sketch "スケッチ19" plane through (0, -66, 0) normal (0, 1, 0) x (-1, 0, 0)
  line L0 (-60.5, 50) -> (-60.5, 41)
  line L1 (-60.5, 41) -> (-39, 41)
  line L2 (-39, 41) -> (-39, 39)
  line L3 (-39, 39) -> (-160.5, 39)
  line L4 (-160.5, 39) -> (-160.5, 41)
  line L5 (-160.5, 41) -> (-139, 41)
  line L6 (-139, 41) -> (-139, 50)
  line L7 (-139, 50) -> (-144.5, 50)
  line L8 (-144.5, 50) -> (-144.5, 53)
  line L9 (-144.5, 53) -> (-150, 53)
  line L10 (-150, 53) -> (-150, 56)
  line L11 (-150, 56) -> (-155.5, 56)
  line L12 (-155.5, 56) -> (-155.5, 59)
  line L13 (-155.5, 59) -> (-161, 59)
  line L14 (-161, 59) -> (-161, 62)
  line L15 (-161, 62) -> (-166.5, 62)
  line L16 (-166.5, 62) -> (-166.5, 65)
  line L17 (-166.5, 65) -> (-172, 65)
  line L18 (-172, 65) -> (-172, 68)
  line L19 (-172, 68) -> (-177.5, 68)
  line L20 (-177.5, 68) -> (-177.5, 71)
  line L21 (-177.5, 71) -> (-183, 71)
  line L22 (-183, 71) -> (-183, 74)
  line L23 (-183, 74) -> (-188.5, 74)
  line L24 (-188.5, 74) -> (-188.5, 77)
  line L25 (-188.5, 77) -> (-194, 77)
  line L26 (-194, 77) -> (-194, 80)
  line L27 (-194, 80) -> (-199.5, 80)
  line L28 (-199.5, 80) -> (-199.5, 3)
  arc A0 (-199.5, 3) -> (-196.5, 0) centre (-196.5, 3) ccw
  line L29 (-196.5, 0) -> (-3, 0)
  arc A1 (-3, 0) -> (0, 3) centre (-3, 3) ccw
  line L30 (0, 3) -> (0, 80)
  line L31 (0, 80) -> (-5.5, 80)
  line L32 (-5.5, 80) -> (-5.5, 77)
  line L33 (-5.5, 77) -> (-11, 77)
  line L34 (-11, 77) -> (-11, 74)
  line L35 (-11, 74) -> (-16.5, 74)
  line L36 (-16.5, 74) -> (-16.5, 71)
  line L37 (-16.5, 71) -> (-22, 71)
  line L38 (-22, 71) -> (-22, 68)
  line L39 (-22, 68) -> (-27.5, 68)
  line L40 (-27.5, 68) -> (-27.5, 65)
  line L41 (-27.5, 65) -> (-33, 65)
  line L42 (-33, 65) -> (-33, 62)
  line L43 (-33, 62) -> (-38.5, 62)
  line L44 (-38.5, 62) -> (-38.5, 59)
  line L45 (-38.5, 59) -> (-44, 59)
  line L46 (-44, 59) -> (-44, 56)
  line L47 (-44, 56) -> (-49.5, 56)
  line L48 (-49.5, 56) -> (-49.5, 53)
  line L49 (-49.5, 53) -> (-55, 53)
  line L50 (-55, 53) -> (-55, 50)
  line L51 (-55, 50) -> (-60.5, 50)
sketch "スケッチ20" plane through (0, -71.5, 0) normal (0, 1, 0) x (-1, 0, 0)
  line L0 (-139, 47) -> (-139, 50)
  line L1 (-139, 50) -> (-144.5, 50)
  line L2 (-144.5, 50) -> (-144.5, 53)
  line L3 (-144.5, 53) -> (-150, 53)
  line L4 (-150, 53) -> (-150, 56)
  line L5 (-150, 56) -> (-155.5, 56)
  line L6 (-155.5, 56) -> (-155.5, 59)
  line L7 (-155.5, 59) -> (-161, 59)
  line L8 (-161, 59) -> (-161, 62)
  line L9 (-161, 62) -> (-166.5, 62)
  line L10 (-166.5, 62) -> (-166.5, 65)
  line L11 (-166.5, 65) -> (-172, 65)
  line L12 (-172, 65) -> (-172, 68)
  line L13 (-172, 68) -> (-177.5, 68)
  line L14 (-177.5, 68) -> (-177.5, 71)
  line L15 (-177.5, 71) -> (-183, 71)
  line L16 (-183, 71) -> (-183, 74)
  line L17 (-183, 74) -> (-188.5, 74)
  line L18 (-188.5, 74) -> (-188.5, 77)
  line L19 (-188.5, 77) -> (-194, 77)
  line L20 (-194, 77) -> (-194, 80)
  line L21 (-194, 80) -> (-199.5, 80)
  line L22 (-199.5, 80) -> (-199.5, 3)
  arc A0 (-199.5, 3) -> (-196.5, 0) centre (-196.5, 3) ccw
  line L23 (-196.5, 0) -> (-3, 0)
  arc A1 (-3, 0) -> (0, 3) centre (-3, 3) ccw
  line L24 (0, 3) -> (0, 80)
  line L25 (0, 80) -> (-5.5, 80)
  line L26 (-5.5, 80) -> (-5.5, 77)
  line L27 (-5.5, 77) -> (-11, 77)
  line L28 (-11, 77) -> (-11, 74)
  line L29 (-11, 74) -> (-16.5, 74)
  line L30 (-16.5, 74) -> (-16.5, 71)
  line L31 (-16.5, 71) -> (-22, 71)
  line L32 (-22, 71) -> (-22, 68)
  line L33 (-22, 68) -> (-27.5, 68)
  line L34 (-27.5, 68) -> (-27.5, 65)
  line L35 (-27.5, 65) -> (-33, 65)
  line L36 (-33, 65) -> (-33, 62)
  line L37 (-33, 62) -> (-38.5, 62)
  line L38 (-38.5, 62) -> (-38.5, 59)
  line L39 (-38.5, 59) -> (-44, 59)
  line L40 (-44, 59) -> (-44, 56)
  line L41 (-44, 56) -> (-49.5, 56)
  line L42 (-49.5, 56) -> (-49.5, 53)
  line L43 (-49.5, 53) -> (-55, 53)
  line L44 (-55, 53) -> (-55, 50)
  line L45 (-55, 50) -> (-60.5, 50)
  line L46 (-60.5, 50) -> (-60.5, 47)
  line L47 (-60.5, 47) -> (-139, 47)